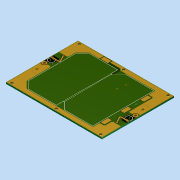
# Autodesk Inventor part: FOX-ME-127-05
Saved by Autodesk Inventor 2014 (Build 180170000, 170)
## iProperties
Created: 2011-02-15
Material: FR4
Document SubType Name: Modeling
Designer: Robert Davis
Mass: 28.2134 g
Surface Area: 181.294 cm^2
Volume: 13.8301 cm^3
Density: 2.04 g/cm^3
Project: PCB
Description: PCB
Part Number: FOX-ME-127-05
Appearance: Gold
Author: Robert Davis
Autodesk Inventor part; units mm, degrees
ref_plane "YZ Plane" through (0, 0, 0) normal (1, 0, 0) x (0, 1, 0)
ref_plane "XZ Plane" through (0, 0, 0) normal (0, 1, 0) x (-1, 0, 0)
ref_plane "XY Plane" through (0, 0, 0) normal (0, 0, 1) x (1, 0, 0)
sketch "Sketch1" plane through (0, 0, 0) normal (0, 0, 1) x (1, 0, 0)
  line L0 (-54, -40.5) -> (54, -40.5)
  line L1 (54, -40.5) -> (54, 40.5)
  line L2 (54, 40.5) -> (-54, 40.5)
  line L3 (-54, 40.5) -> (-54, -40.5)
  point P0 (0, 0)
  dimension "d0" = 108
  dimension "d1" = 81
  dimension "d2" = 40.5
  dimension "d3" = 54
  constraints: 8 end point, 2 horizontal, 2 vertical
  measures "d0" distance of L1.end L2.end
  measures "d1" distance of L0.end L1.end
  measures "d2" distance from line of point (0, 0) L2
  measures "d3" distance from line of L1 point (0, 0)
extrude "Extrusion1" add sketch "Sketch1" along normal blind 1.5875
hole "Hole2" at (50, -38, 1.5875) direction (0, 0, -1) diameter 2.6924 end through all
mirror "Mirror1" about plane through (0, 0, 0) normal (0, 1, 0) of "Hole2"
hole "Hole3" [suppressed]
hole "Hole4" [suppressed]
mirror "Mirror2" about plane through (0, 0, 0) normal (1, 0, 0) of "Hole2", "Mirror1"
hole "Hole5" at (0, -38, 1.5875) direction (0, 0, -1) diameter 2.6924 end through all
mirror "Mirror3" about plane through (0, 0, 0) normal (0, 1, 0) of "Hole5"
hole "Hole6" at (51.25, 0, 0) direction (0, 0, 1) diameter 2.6924 end through all
mirror "Mirror4" about plane through (0, 0, 0) normal (1, 0, 0) of "Hole6"
hole "Hole_spring" at (-47.6, 17.5, 1.5875) direction (0, 0, -1) diameter 0.5 end through all
sketch "Sketch3" plane through (0, 0, 1.5875) normal (0, 0, 1) x (1, 0, 0)
  line L0 (-54, -40.5) -> (-54, 40.5) projected
  line L1 (-54, 40.5) -> (54, 40.5) projected
  line L2 (-47.6, 9.8024) -> (-47.6, -15.4623) construction
  circle A0 centre (-45.6, 3.5) radius 0.25
  circle A1 centre (-49.6, -10.0207) radius 0.25
  point P0 (0, 0)
  point P1 (-46.1616, -3.6859)
  dimension "d243" = 6.4
  dimension "d244" = 2
  dimension "d245" = 2
  dimension "d246" = 14.1
  dimension "d247" = 0.5
  dimension "d248" = 37
  constraints: 2 centre point, 2 end point, 1 equal radius
  measures "d243" distance between parallel lines of L0 L2
  measures "d244" distance from line of L2 A1.centre
  measures "d245" distance from line of L2 A0.centre
  measures "d246" distance of A1.centre A0.centre
  measures "d247" diameter of A1
  measures "d248" distance from line of L1 A0.centre
extrude "Holes_resistor" cut sketch "Sketch3" against normal through all
hole "Hole_via" at (-50, 9, 1.5875) direction (0, 0, -1) diameter 0.5 end through all
hole "Hole_spring_2" at (47.6, -17.5, 1.5875) direction (0, 0, -1) diameter 0.5 end through all
sketch "Sketch5" plane through (0, 0, 1.5875) normal (0, 0, 1) x (1, 0, 0)
  line L0 (54, -40.5) -> (-54, -40.5) projected
  line L1 (54, 40.5) -> (54, -40.5) projected
  line L2 (47.6, -11.3866) -> (47.6, 14.8402) construction
  circle A0 centre (49.6, 10.0207) radius 0.25
  circle A1 centre (45.6, -3.5) radius 0.25
  point P0 (0, 0)
  dimension "d271" = 6.4
  dimension "d272" = 2
  dimension "d273" = 2
  dimension "d274" = 0.5
  dimension "d275" = 14.1
  dimension "d276" = 37
  constraints: 2 centre point, 2 end point, 1 equal radius
  measures "d271" distance between parallel lines of L2 L1
  measures "d272" distance from line of L2 A0.centre
  measures "d273" distance from line of L2 A1.centre
  measures "d274" diameter of A0
  measures "d275" distance of A1.centre A0.centre
  measures "d276" distance from line of L0 A1.centre
extrude "Holes_resistor2" cut sketch "Sketch5" against normal through all
hole "Hole_via2" at (50, -9, 1.5875) direction (0, 0, -1) diameter 0.5 end through all
hole "Hole26" at (-52.5, 10.25, 1.5875) direction (0, 0, -1) diameter 0.6 end through all
hole "Hole27" at (52.5, -10.25, 1.5875) direction (0, 0, -1) diameter 0.6 end through all
sketch "Sketch8" plane through (0, 0, 1.5875) normal (0, 0, 1) x (1, 0, 0)
  line L0 (-54, -40.5) -> (-54, 40.5) projected
  line L1 (54, -40.5) -> (-54, -40.5) projected
  line L2 (54, 40.5) -> (54, -40.5) projected
  line L3 (-54, 40.5) -> (54, 40.5) projected
  line L4 (54.0603, -40.4195) -> (-54, -40.5) construction
  line L5 (-54, -40.5) -> (-54.0603, 40.4195) construction
  line L6 (-54.0603, 40.4195) -> (54, 40.5) construction
  line L7 (54, 40.5) -> (54.0603, -40.4195) construction
  point P0 (0, 0)
  constraints: 4 point on line, 2 other
decal "Decal3"
sketch "Sketch9" plane through (0, 0, 0) normal (0, 0, -1) x (-1, 0, 0)
  line L0 (54, -40.5) -> (-54, -40.5) projected
  line L1 (54, 40.5) -> (54, -40.5) projected
  line L2 (-54, 40.5) -> (54, 40.5) projected
  line L3 (-54, -40.5) -> (-54, 40.5) projected
  line L4 (54.0603, -40.4195) -> (-54, -40.5) construction
  line L5 (-54, -40.5) -> (-54.0603, 40.4195) construction
  line L6 (-54.0603, 40.4195) -> (54, 40.5) construction
  line L7 (54, 40.5) -> (54.0603, -40.4195) construction
  point P0 (0, 0)
  constraints: 4 point on line, 2 other
decal "Decal4"
equation "\"d283\" = d253"
equation "\"d253\" = 0.5"
body "Solid1"
